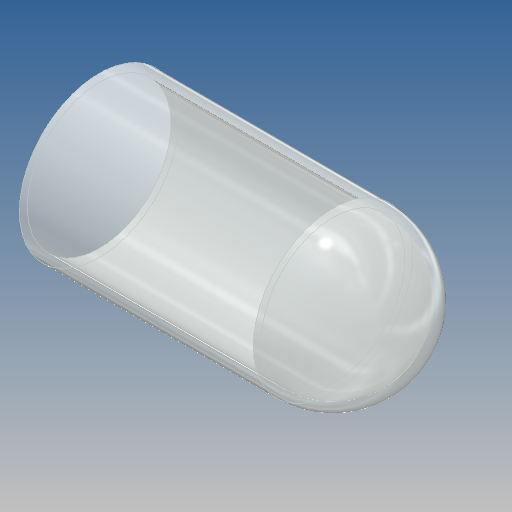
# Autodesk Inventor part: Außenkolben
Saved by Autodesk Inventor 2018 (Build 220112000, 112)
## iProperties
Created: 2018-10-23
Part Number: Außenkolben
Material: Glas
Document SubType Name: Modeling
Designer: M.Knabel
Density: 2.18 g/cm^3
Appearance: Klar
Mass: 13.8521 g
Surface Area: 91.9846 cm^2
Volume: 6.35415 cm^3
Author: M.Knabel
Autodesk Inventor part; units mm, degrees
ref_plane "YZ Plane" through (0, 0, 0) normal (1, 0, 0) x (0, 1, 0)
ref_plane "XZ Plane" through (0, 0, 0) normal (0, 1, 0) x (-1, 0, 0)
ref_plane "XY Plane" through (0, 0, 0) normal (0, 0, 1) x (1, 0, 0)
sketch "Skizze1" plane through (0, 0, 0) normal (0, 0, 1) x (1, 0, 0)
  line L0 (0, -3.3799) -> (0, 20.2794) projected
  line L1 (-11.5799, 0) -> (69.4794, 0) projected
  line L2 (0, 12.6) -> (41, 12.6)
  line L3 (0, 12.6) -> (0, 14)
  line L4 (0, 14) -> (41, 14)
  arc A0 (53.6, 0) -> (41, 12.6) centre (41, 0) ccw
  arc A1 (55, 0) -> (41, 14) centre (41, 0) ccw
  line L5 (53.6, 0) -> (55, 0)
  point P0 (0, 0)
  dimension "d0" = 14
  dimension "d1" = 1.4
  dimension "d2" = 28
  dimension "d3" = 55
  constraints: 8 end point, 4 point on circle, 4 point on line, 2 centre point, 2 horizontal, 2 tangent, 1 collinear, 1 concentric
  measures "d0" radius of A1
  measures "d1" distance between parallel lines of L4 L2
  measures "d2" diameter of L4 L1
  measures "d3" distance from line of L0 L5.end
revolve "Umdrehung1" add sketch "Skizze1" angle 360 about axis through (-10, 0, 0) along (1, 0, 0) contours L0 L4 A1 L1 A0 L2
